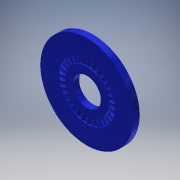
# Autodesk Inventor part: wheel hub
Saved by Autodesk Inventor 2017 (Build 210142000, 142)
## iProperties
Created: 2017-11-23
Part Number: wheel hub
Material: ABS Plastic
Document SubType Name: Modeling
Designer: prakh
Density: 1.06 g/cm^3
Appearance: Blue - Wall Paint - Glossy
Author: prakh
Autodesk Inventor part; units mm, degrees
ref_plane "YZ Plane" through (0, 0, 0) normal (1, 0, 0) x (0, 1, 0)
ref_plane "XZ Plane" through (0, 0, 0) normal (0, 1, 0) x (-1, 0, 0)
ref_plane "XY Plane" through (0, 0, 0) normal (0, 0, 1) x (1, 0, 0)
sketch "Sketch1" plane through (0, 0, 0) normal (0, 0, 1) x (1, 0, 0)
  circle A0 centre (0, 0) radius 47.625
  line L0 (2.7496, 4.7625) -> (5.4993, 0)
  line L1 (5.4993, 0) -> (2.7496, -4.7625)
  line L2 (2.7496, -4.7625) -> (-2.7496, -4.7625)
  line L3 (-2.7496, -4.7625) -> (-5.4993, 0)
  line L4 (-5.4993, 0) -> (-2.7496, 4.7625)
  line L5 (-2.7496, 4.7625) -> (2.7496, 4.7625)
  circle A1 centre (0, 0) radius 14.2875
  dimension "d0" = 95.25
  dimension "d3" = 9.525
  dimension "d22" = 28.575
  constraints: 12 end point, 3 coincident, 2 centre point, 13 other
  measures "d0" diameter of A0
  measures "d3" distance between parallel lines of L5 L2
  measures "d22" diameter of A1
extrude "Extrusion1" add sketch "Sketch1" along normal blind 3.175 contours A0
sketch "Sketch3" plane through (0, 0, 3.175) normal (0, 0, 1) x (1, 0, 0)
  circle A0 centre (0, 0) radius 22.225
  circle A1 centre (0, 0) radius 28.575
  dimension "d4" = 44.45
  dimension "d6" = 6.35
  constraints: 2 centre point, 2 coincident
  measures "d4" diameter of A0
  measures "d6" radial gap between concentric circles of A1 A0
extrude "Extrusion2" add sketch "Sketch3" along normal blind 3.175
sketch "Sketch4" plane through (0, 0, 0) normal (1, 0, 0) x (0, 1, 0)
  line L0 (28.575, 6.35) -> (-28.575, 6.35) projected
  arc A0 (-2.7496, 6.35) -> (2.7496, 6.35) centre (0, 7.9375) ccw
  point P0 (0, 0)
  dimension "d9" = 3.175
  dimension "d10" = 1.5875
  constraints: 2 point on circle, 2 point on line, 1 centre point, 1 vertical alignment
  measures "d9" radius of A0
  measures "d10" distance from line of A0.centre L0
extrude "Extrusion3" cut sketch "Sketch4" along normal blind 31.75
pattern_circular "Circular Pattern1" count 30 over 360 about axis through (0, 0, -10) along (0, 0, 1) of "Extrusion3"
sketch "Sketch5" plane through (0, 0, 3.175) normal (0, 0, 1) x (1, 0, 0)
  circle A0 centre (0, 0) radius 22.225
  circle A1 centre (0, 0) radius 19.05
  circle A2 centre (0, 0) radius 28.575
  circle A3 centre (0, 0) radius 31.75
  circle A4 centre (0, 0) radius 47.625 projected
  circle A5 centre (0, 0) radius 22.225 projected
  circle A6 centre (0, 0) radius 14.2875 projected
  dimension "d16" = 3.175
  dimension "d17" = 44.45
  dimension "d18" = 57.15
  dimension "d19" = 3.175
  constraints: 4 centre point, 4 coincident
  measures "d16" radial gap between concentric circles of A1 A0
  measures "d17" diameter of A0
  measures "d18" diameter of A2
  measures "d19" radial gap between concentric circles of A2 A3
extrude "Extrusion4" add sketch "Sketch5" along normal up to surface (3.175 mm away) contours A0 | A1 | A3 | A4
equation "\"d16\" = d19"
body "Solid1"
